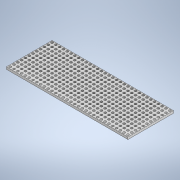
# Autodesk Inventor part: TamiyaUniversalPlate60-160
Saved by Autodesk Inventor 2022 (Build 260153000, 153)
## iProperties
Created: 2021-07-08
Part Number: TamiyaUniversalPlate60-160
Material: 一般
Document SubType Name: Modeling
Designer: ken
Density: 1 g/cm^3
Appearance: 既定
Author: ken
Autodesk Inventor part; units mm, degrees
ref_plane "YZ Plane" through (0, 0, 0) normal (1, 0, 0) x (0, 1, 0)
ref_plane "XZ Plane" through (0, 0, 0) normal (0, 1, 0) x (-1, 0, 0)
ref_plane "XY Plane" through (0, 0, 0) normal (0, 0, 1) x (1, 0, 0)
sketch "スケッチ1" plane through (0, 0, 0) normal (0, 1, 0) x (-1, 0, 0)
  line L0 (0, 0) -> (160, 0)
  line L1 (160, 0) -> (160, -60)
  line L2 (160, -60) -> (0, -60)
  line L3 (0, -60) -> (0, 0)
  dimension "d0" = 160
  dimension "d1" = 60
  constraints: 8 end point, 2 parallel, 1 horizontal, 1 perpendicular
  measures "d0" distance of L1.end L2.end
  measures "d1" distance of L0.end L1.end
extrude "押し出し1" add sketch "スケッチ1" along normal blind 3
sketch "スケッチ2" plane through (0, 3, 0) normal (0, 1, 0) x (1, 0, 0)
  line L0 (-160, 60) -> (-160, 0) projected
  line L1 (-160, 0) -> (0, 0) projected
  line L2 (0, 60) -> (-160, 60) projected
  line L3 (0, 0) -> (0, 60) projected
  point P0 (-77.5, 2.5)
  point P1 (-77.5, 7.5)
  point P2 (-77.5, 12.5)
  point P3 (-77.5, 17.5)
  point P4 (-77.5, 22.5)
  point P5 (-77.5, 27.5)
  point P6 (-77.5, 32.5)
  point P7 (-77.5, 37.5)
  point P8 (-77.5, 47.5)
  point P9 (-77.5, 42.5)
  point P10 (-77.5, 52.5)
  point P11 (-77.5, 57.5)
  point P12 (-72.5, 2.5)
  point P13 (-72.5, 7.5)
  point P14 (-72.5, 12.5)
  point P15 (-72.5, 17.5)
  point P16 (-72.5, 22.5)
  point P17 (-72.5, 27.5)
  point P18 (-72.5, 32.5)
  point P19 (-72.5, 37.5)
  point P20 (-72.5, 47.5)
  point P21 (-72.5, 42.5)
  point P22 (-72.5, 52.5)
  point P23 (-72.5, 57.5)
  point P24 (-67.5, 2.5)
  point P25 (-67.5, 7.5)
  point P26 (-67.5, 12.5)
  point P27 (-67.5, 17.5)
  point P28 (-67.5, 22.5)
  point P29 (-67.5, 27.5)
  point P30 (-67.5, 32.5)
  point P31 (-67.5, 37.5)
  point P32 (-67.5, 47.5)
  point P33 (-67.5, 42.5)
  point P34 (-67.5, 52.5)
  point P35 (-67.5, 57.5)
  point P36 (-62.5, 2.5)
  point P37 (-62.5, 7.5)
  point P38 (-62.5, 12.5)
  point P39 (-62.5, 17.5)
  point P40 (-62.5, 22.5)
  point P41 (-62.5, 27.5)
  point P42 (-62.5, 32.5)
  point P43 (-62.5, 37.5)
  point P44 (-62.5, 47.5)
  point P45 (-62.5, 42.5)
  point P46 (-62.5, 52.5)
  point P47 (-62.5, 57.5)
  point P48 (-57.5, 2.5)
  point P49 (-57.5, 7.5)
  point P50 (-57.5, 12.5)
  point P51 (-57.5, 17.5)
  point P52 (-57.5, 22.5)
  point P53 (-57.5, 27.5)
  point P54 (-57.5, 32.5)
  point P55 (-57.5, 37.5)
  point P56 (-57.5, 47.5)
  point P57 (-57.5, 42.5)
  point P58 (-57.5, 52.5)
  point P59 (-57.5, 57.5)
  point P60 (-52.5, 57.5)
  point P61 (-52.5, 52.5)
  point P62 (-52.5, 42.5)
  point P63 (-52.5, 47.5)
  point P64 (-52.5, 37.5)
  point P65 (-52.5, 32.5)
  point P66 (-52.5, 27.5)
  point P67 (-52.5, 22.5)
  point P68 (-52.5, 17.5)
  point P69 (-52.5, 12.5)
  point P70 (-52.5, 7.5)
  point P71 (-52.5, 2.5)
  point P72 (-47.5, 57.5)
  point P73 (-47.5, 52.5)
  point P74 (-47.5, 42.5)
  point P75 (-47.5, 47.5)
  point P76 (-47.5, 37.5)
  point P77 (-47.5, 32.5)
  point P78 (-47.5, 27.5)
  point P79 (-47.5, 22.5)
  point P80 (-47.5, 17.5)
  point P81 (-47.5, 12.5)
  point P82 (-47.5, 7.5)
  point P83 (-47.5, 2.5)
  point P84 (-42.5, 57.5)
  point P85 (-42.5, 52.5)
  point P86 (-42.5, 42.5)
  point P87 (-42.5, 47.5)
  point P88 (-42.5, 37.5)
  point P89 (-42.5, 32.5)
  point P90 (-42.5, 27.5)
  point P91 (-42.5, 22.5)
  point P92 (-42.5, 17.5)
  point P93 (-42.5, 12.5)
  point P94 (-42.5, 7.5)
  point P95 (-42.5, 2.5)
  point P96 (-37.5, 2.5)
  point P97 (-37.5, 7.5)
  point P98 (-37.5, 12.5)
  point P99 (-37.5, 17.5)
  point P100 (-37.5, 22.5)
  point P101 (-37.5, 27.5)
  point P102 (-37.5, 32.5)
  point P103 (-37.5, 37.5)
  point P104 (-37.5, 47.5)
  point P105 (-37.5, 42.5)
  point P106 (-37.5, 52.5)
  point P107 (-37.5, 57.5)
  point P108 (-32.5, 57.5)
  point P109 (-32.5, 52.5)
  point P110 (-32.5, 42.5)
  point P111 (-32.5, 47.5)
  point P112 (-32.5, 37.5)
  point P113 (-32.5, 32.5)
  point P114 (-32.5, 27.5)
  point P115 (-32.5, 22.5)
  point P116 (-32.5, 17.5)
  point P117 (-32.5, 12.5)
  point P118 (-32.5, 7.5)
  point P119 (-32.5, 2.5)
  point P120 (-27.5, 57.5)
  point P121 (-27.5, 52.5)
  point P122 (-27.5, 42.5)
  point P123 (-27.5, 47.5)
  point P124 (-27.5, 37.5)
  point P125 (-27.5, 32.5)
  point P126 (-27.5, 27.5)
  point P127 (-27.5, 22.5)
  point P128 (-27.5, 17.5)
  point P129 (-27.5, 12.5)
  point P130 (-27.5, 7.5)
  point P131 (-27.5, 2.5)
  point P132 (-22.5, 57.5)
  point P133 (-22.5, 52.5)
  point P134 (-22.5, 42.5)
  point P135 (-22.5, 47.5)
  point P136 (-22.5, 37.5)
  point P137 (-22.5, 32.5)
  point P138 (-22.5, 27.5)
  point P139 (-22.5, 22.5)
  point P140 (-22.5, 17.5)
  point P141 (-22.5, 12.5)
  point P142 (-22.5, 7.5)
  point P143 (-22.5, 2.5)
  point P144 (-17.5, 2.5)
  point P145 (-17.5, 7.5)
  point P146 (-17.5, 12.5)
  point P147 (-17.5, 17.5)
  point P148 (-17.5, 22.5)
  point P149 (-17.5, 27.5)
  point P150 (-17.5, 32.5)
  point P151 (-17.5, 37.5)
  point P152 (-17.5, 47.5)
  point P153 (-17.5, 42.5)
  point P154 (-17.5, 52.5)
  point P155 (-17.5, 57.5)
  point P156 (-12.5, 57.5)
  point P157 (-12.5, 52.5)
  point P158 (-12.5, 42.5)
  point P159 (-12.5, 47.5)
  point P160 (-12.5, 37.5)
  point P161 (-12.5, 32.5)
  point P162 (-12.5, 27.5)
  point P163 (-12.5, 22.5)
  point P164 (-12.5, 17.5)
  point P165 (-12.5, 12.5)
  point P166 (-12.5, 7.5)
  point P167 (-12.5, 2.5)
  point P168 (-7.5, 57.5)
  point P169 (-7.5, 52.5)
  point P170 (-7.5, 42.5)
  point P171 (-7.5, 47.5)
  point P172 (-7.5, 37.5)
  point P173 (-7.5, 32.5)
  point P174 (-7.5, 27.5)
  point P175 (-7.5, 22.5)
  point P176 (-7.5, 17.5)
  point P177 (-7.5, 12.5)
  point P178 (-7.5, 7.5)
  point P179 (-7.5, 2.5)
  point P180 (-2.5, 57.5)
  point P181 (-2.5, 52.5)
  point P182 (-2.5, 42.5)
  point P183 (-2.5, 47.5)
  point P184 (-2.5, 37.5)
  point P185 (-2.5, 32.5)
  point P186 (-2.5, 27.5)
  point P187 (-2.5, 22.5)
  point P188 (-2.5, 17.5)
  point P189 (-2.5, 12.5)
  point P190 (-2.5, 7.5)
  point P191 (-2.5, 2.5)
  point P192 (-157.5, 2.5)
  point P193 (-157.5, 7.5)
  point P194 (-157.5, 12.5)
  point P195 (-157.5, 17.5)
  point P196 (-157.5, 22.5)
  point P197 (-157.5, 27.5)
  point P198 (-157.5, 32.5)
  point P199 (-157.5, 37.5)
  dimension "d4" = 5
  dimension "d5" = 2.5
  dimension "d6" = 5
  dimension "d7" = 5
  dimension "d8" = 5
  dimension "d9" = 5
  dimension "d10" = 5
  dimension "d11" = 5
  dimension "d12" = 5
  dimension "d13" = 5
  dimension "d14" = 5
  dimension "d15" = 5
  dimension "d16" = 2.5
  dimension "d17" = 2.5
  dimension "d18" = 5
  dimension "d19" = 5
  dimension "d20" = 5
  dimension "d21" = 5
  dimension "d22" = 5
  dimension "d23" = 5
  dimension "d24" = 5
  dimension "d25" = 5
  dimension "d26" = 5
  dimension "d27" = 5
  dimension "d28" = 5
  dimension "d29" = 5
  dimension "d30" = 5
  dimension "d31" = 5
  dimension "d32" = 5
  dimension "d33" = 5
  dimension "d34" = 5
  dimension "d35" = 5
  dimension "d36" = 5
  dimension "d37" = 5
  dimension "d38" = 5
  dimension "d39" = 5
  dimension "d40" = 5
  dimension "d41" = 5
  dimension "d42" = 5
  dimension "d43" = 5
  dimension "d44" = 5
  dimension "d45" = 5
  dimension "d46" = 5
  dimension "d47" = 5
  dimension "d48" = 5
  dimension "d49" = 5
  dimension "d50" = 5
  dimension "d51" = 5
  dimension "d52" = 5
  dimension "d53" = 5
  dimension "d54" = 5
  dimension "d55" = 5
  dimension "d56" = 5
  dimension "d57" = 5
  dimension "d58" = 5
  dimension "d59" = 5
  dimension "d60" = 5
  dimension "d61" = 5
  dimension "d62" = 5
  dimension "d63" = 5
  dimension "d64" = 5
  dimension "d65" = 5
  dimension "d66" = 5
  dimension "d67" = 5
  constraints: 352 vertical alignment, 24 horizontal alignment
  measures "d4" distance of point (-77.5, 2.5) point (-77.5, 7.5)
  measures "d6" distance of point (-77.5, 7.5) point (-77.5, 12.5)
  measures "d7" distance of point (-77.5, 12.5) point (-77.5, 17.5)
  measures "d8" distance of point (-77.5, 17.5) point (-77.5, 22.5)
  measures "d9" distance of point (-77.5, 22.5) point (-77.5, 27.5)
  measures "d10" distance of point (-77.5, 27.5) point (-77.5, 32.5)
  measures "d11" distance of point (-77.5, 37.5) point (-77.5, 32.5)
  measures "d12" distance of point (-77.5, 42.5) point (-77.5, 37.5)
  measures "d13" distance of point (-77.5, 47.5) point (-77.5, 42.5)
  measures "d14" distance of point (-77.5, 52.5) point (-77.5, 47.5)
  measures "d15" distance of point (-77.5, 57.5) point (-77.5, 52.5)
  measures "d16" distance from line of L1 point (-77.5, 2.5)
  measures "d17" distance from line of L2 point (-77.5, 57.5)
  measures "d18" distance of point (-72.5, 2.5) point (-72.5, 7.5)
  measures "d19" distance of point (-72.5, 7.5) point (-72.5, 12.5)
  measures "d20" distance of point (-72.5, 12.5) point (-72.5, 17.5)
  measures "d21" distance of point (-72.5, 17.5) point (-72.5, 22.5)
  measures "d22" distance of point (-72.5, 22.5) point (-72.5, 27.5)
  measures "d23" distance of point (-72.5, 27.5) point (-72.5, 32.5)
  measures "d24" distance of point (-72.5, 37.5) point (-72.5, 32.5)
  measures "d25" distance of point (-72.5, 42.5) point (-72.5, 37.5)
  measures "d26" distance of point (-72.5, 47.5) point (-72.5, 42.5)
  measures "d27" distance of point (-72.5, 52.5) point (-72.5, 47.5)
  measures "d28" distance of point (-72.5, 57.5) point (-72.5, 52.5)
  measures "d29" distance of point (-67.5, 2.5) point (-67.5, 7.5)
  measures "d30" distance of point (-67.5, 7.5) point (-67.5, 12.5)
  measures "d31" distance of point (-67.5, 12.5) point (-67.5, 17.5)
  measures "d32" distance of point (-67.5, 17.5) point (-67.5, 22.5)
  measures "d33" distance of point (-67.5, 22.5) point (-67.5, 27.5)
  measures "d34" distance of point (-67.5, 27.5) point (-67.5, 32.5)
  measures "d35" distance of point (-67.5, 37.5) point (-67.5, 32.5)
  measures "d36" distance of point (-67.5, 42.5) point (-67.5, 37.5)
  measures "d37" distance of point (-67.5, 47.5) point (-67.5, 42.5)
  measures "d38" distance of point (-67.5, 52.5) point (-67.5, 47.5)
  measures "d39" distance of point (-67.5, 57.5) point (-67.5, 52.5)
  measures "d40" distance of point (-62.5, 2.5) point (-62.5, 7.5)
  measures "d41" distance of point (-62.5, 7.5) point (-62.5, 12.5)
  measures "d42" distance of point (-62.5, 12.5) point (-62.5, 17.5)
  measures "d43" distance of point (-62.5, 17.5) point (-62.5, 22.5)
  measures "d44" distance of point (-62.5, 22.5) point (-62.5, 27.5)
  measures "d45" distance of point (-62.5, 27.5) point (-62.5, 32.5)
  measures "d46" distance of point (-62.5, 37.5) point (-62.5, 32.5)
  measures "d47" distance of point (-62.5, 42.5) point (-62.5, 37.5)
  measures "d48" distance of point (-62.5, 47.5) point (-62.5, 42.5)
  measures "d49" distance of point (-62.5, 52.5) point (-62.5, 47.5)
  measures "d50" distance of point (-62.5, 57.5) point (-62.5, 52.5)
  measures "d51" distance of point (-77.5, 2.5) point (-72.5, 2.5)
  measures "d52" distance of point (-72.5, 2.5) point (-67.5, 2.5)
  measures "d53" distance of point (-67.5, 2.5) point (-62.5, 2.5)
  measures "d54" distance of point (-57.5, 2.5) point (-57.5, 7.5)
  measures "d55" distance of point (-57.5, 7.5) point (-57.5, 12.5)
  measures "d56" distance of point (-57.5, 12.5) point (-57.5, 17.5)
  measures "d57" distance of point (-57.5, 17.5) point (-57.5, 22.5)
  measures "d58" distance of point (-57.5, 22.5) point (-57.5, 27.5)
  measures "d59" distance of point (-57.5, 27.5) point (-57.5, 32.5)
  measures "d60" distance of point (-57.5, 37.5) point (-57.5, 32.5)
  measures "d61" distance of point (-57.5, 42.5) point (-57.5, 37.5)
  measures "d62" distance of point (-57.5, 47.5) point (-57.5, 42.5)
  measures "d63" distance of point (-57.5, 52.5) point (-57.5, 47.5)
  measures "d64" distance of point (-57.5, 57.5) point (-57.5, 52.5)
  measures "d65" distance of point (-52.5, 2.5) point (-52.5, 7.5)
  measures "d66" distance of point (-52.5, 7.5) point (-52.5, 12.5)
  measures "d67" distance of point (-52.5, 12.5) point (-52.5, 17.5)
hole "穴1" at (-157.5, 3, -2.5) at (-157.5, 3, -7.5) at (-157.5, 3, -12.5) at (-157.5, 3, -17.5) at (-157.5, 3, -22.5) at (-157.5, 3, -27.5) at (-157.5, 3, -32.5) at (-157.5, 3, -37.5) at (-157.5, 3, -47.5) at (-157.5, 3, -42.5) at (-157.5, 3, -52.5) at (-157.5, 3, -57.5) at (-152.5, 3, -57.5) at (-152.5, 3, -52.5) at (-152.5, 3, -42.5) at (-152.5, 3, -47.5) at (-152.5, 3, -37.5) at (-152.5, 3, -32.5) at (-152.5, 3, -27.5) at (-152.5, 3, -22.5) at (-152.5, 3, -17.5) at (-152.5, 3, -12.5) at (-152.5, 3, -7.5) at (-152.5, 3, -2.5) at (-147.5, 3, -57.5) at (-147.5, 3, -52.5) at (-147.5, 3, -42.5) at (-147.5, 3, -47.5) at (-147.5, 3, -37.5) at (-147.5, 3, -32.5) at (-147.5, 3, -27.5) at (-147.5, 3, -22.5) at (-147.5, 3, -17.5) at (-147.5, 3, -12.5) at (-147.5, 3, -7.5) at (-147.5, 3, -2.5) at (-142.5, 3, -57.5) at (-142.5, 3, -52.5) at (-142.5, 3, -42.5) at (-142.5, 3, -47.5) at (-142.5, 3, -37.5) at (-142.5, 3, -32.5) at (-142.5, 3, -27.5) at (-142.5, 3, -22.5) at (-142.5, 3, -17.5) at (-142.5, 3, -12.5) at (-142.5, 3, -7.5) at (-142.5, 3, -2.5) at (-122.5, 3, -2.5) at (-122.5, 3, -7.5) direction (0, -1, 0) diameter 3 depth 3 and at (-122.5, 3, -12.5) (-122.5, 3, -17.5) (-122.5, 3, -22.5) (-122.5, 3, -27.5) (-122.5, 3, -32.5) (-122.5, 3, -37.5) (-122.5, 3, -47.5) (-122.5, 3, -42.5) (-122.5, 3, -52.5) (-122.5, 3, -57.5) (-127.5, 3, -2.5) (-127.5, 3, -7.5) (-127.5, 3, -12.5) (-127.5, 3, -17.5) (-127.5, 3, -22.5) (-127.5, 3, -27.5) (-127.5, 3, -32.5) (-127.5, 3, -37.5) (-127.5, 3, -47.5) (-127.5, 3, -42.5) (-127.5, 3, -52.5) (-127.5, 3, -57.5) (-132.5, 3, -2.5) (-132.5, 3, -7.5) (-132.5, 3, -12.5) (-132.5, 3, -17.5) (-132.5, 3, -22.5) (-132.5, 3, -27.5) (-132.5, 3, -32.5) (-132.5, 3, -37.5) (-132.5, 3, -47.5) (-132.5, 3, -42.5) (-132.5, 3, -52.5) (-132.5, 3, -57.5) (-137.5, 3, -57.5) (-137.5, 3, -52.5) (-137.5, 3, -42.5) (-137.5, 3, -47.5) (-137.5, 3, -37.5) (-137.5, 3, -32.5) (-137.5, 3, -27.5) (-137.5, 3, -22.5) (-137.5, 3, -17.5) (-137.5, 3, -12.5) (-137.5, 3, -7.5) (-137.5, 3, -2.5) (-102.5, 3, -2.5) (-102.5, 3, -7.5) (-102.5, 3, -12.5) (-102.5, 3, -17.5) (-102.5, 3, -22.5) (-102.5, 3, -27.5) (-102.5, 3, -32.5) (-102.5, 3, -37.5) (-102.5, 3, -47.5) (-102.5, 3, -42.5) (-102.5, 3, -52.5) (-102.5, 3, -57.5) (-107.5, 3, -2.5) (-107.5, 3, -7.5) (-107.5, 3, -12.5) (-107.5, 3, -17.5) (-107.5, 3, -22.5) (-107.5, 3, -27.5) (-107.5, 3, -32.5) (-107.5, 3, -37.5) (-107.5, 3, -47.5) (-107.5, 3, -42.5) (-107.5, 3, -52.5) (-107.5, 3, -57.5) (-112.5, 3, -2.5) (-112.5, 3, -7.5) (-112.5, 3, -12.5) (-112.5, 3, -17.5) (-112.5, 3, -22.5) (-112.5, 3, -27.5) (-112.5, 3, -32.5) (-112.5, 3, -37.5) (-112.5, 3, -47.5) (-112.5, 3, -42.5) (-112.5, 3, -52.5) (-112.5, 3, -57.5) (-117.5, 3, -57.5) (-117.5, 3, -52.5) (-117.5, 3, -42.5) (-117.5, 3, -47.5) (-117.5, 3, -37.5) (-117.5, 3, -32.5) (-117.5, 3, -27.5) (-117.5, 3, -22.5) (-117.5, 3, -17.5) (-117.5, 3, -12.5) (-117.5, 3, -7.5) (-117.5, 3, -2.5) (-82.5, 3, -2.5) (-82.5, 3, -7.5) (-82.5, 3, -12.5) (-82.5, 3, -17.5) (-82.5, 3, -22.5) (-82.5, 3, -27.5) (-82.5, 3, -32.5) (-82.5, 3, -37.5) (-82.5, 3, -47.5) (-82.5, 3, -42.5) (-82.5, 3, -52.5) (-82.5, 3, -57.5) (-87.5, 3, -2.5) (-87.5, 3, -7.5) (-87.5, 3, -12.5) (-87.5, 3, -17.5) (-87.5, 3, -22.5) (-87.5, 3, -27.5) (-87.5, 3, -32.5) (-87.5, 3, -37.5) (-87.5, 3, -47.5) (-87.5, 3, -42.5) (-87.5, 3, -52.5) (-87.5, 3, -57.5) (-92.5, 3, -2.5) (-92.5, 3, -7.5) (-92.5, 3, -12.5) (-92.5, 3, -17.5) (-92.5, 3, -22.5) (-92.5, 3, -27.5) (-92.5, 3, -32.5) (-92.5, 3, -37.5) (-92.5, 3, -47.5) (-92.5, 3, -42.5) (-92.5, 3, -52.5) (-92.5, 3, -57.5) (-97.5, 3, -57.5) (-97.5, 3, -52.5) (-97.5, 3, -42.5) (-97.5, 3, -47.5) (-97.5, 3, -37.5) (-97.5, 3, -32.5) (-97.5, 3, -27.5) (-97.5, 3, -22.5) (-97.5, 3, -17.5) (-97.5, 3, -12.5) (-97.5, 3, -7.5) (-97.5, 3, -2.5) (-17.5, 3, -2.5) (-17.5, 3, -7.5) (-17.5, 3, -12.5) (-17.5, 3, -17.5) (-17.5, 3, -22.5) (-17.5, 3, -27.5) (-17.5, 3, -32.5) (-17.5, 3, -37.5) (-17.5, 3, -47.5) (-17.5, 3, -42.5) (-17.5, 3, -52.5) (-17.5, 3, -57.5) (-12.5, 3, -57.5) (-12.5, 3, -52.5) (-12.5, 3, -42.5) (-12.5, 3, -47.5) (-12.5, 3, -37.5) (-12.5, 3, -32.5) (-12.5, 3, -27.5) (-12.5, 3, -22.5) (-12.5, 3, -17.5) (-12.5, 3, -12.5) (-12.5, 3, -7.5) (-12.5, 3, -2.5) (-7.5, 3, -57.5) (-7.5, 3, -52.5) (-7.5, 3, -42.5) (-7.5, 3, -47.5) (-7.5, 3, -37.5) (-7.5, 3, -32.5) (-7.5, 3, -27.5) (-7.5, 3, -22.5) (-7.5, 3, -17.5) (-7.5, 3, -12.5) (-7.5, 3, -7.5) (-7.5, 3, -2.5) (-2.5, 3, -57.5) (-2.5, 3, -52.5) (-2.5, 3, -42.5) (-2.5, 3, -47.5) (-2.5, 3, -37.5) (-2.5, 3, -32.5) (-2.5, 3, -27.5) (-2.5, 3, -22.5) (-2.5, 3, -17.5) (-2.5, 3, -12.5) (-2.5, 3, -7.5) (-2.5, 3, -2.5) (-37.5, 3, -2.5) (-37.5, 3, -7.5) (-37.5, 3, -12.5) (-37.5, 3, -17.5) (-37.5, 3, -22.5) (-37.5, 3, -27.5) (-37.5, 3, -32.5) (-37.5, 3, -37.5) (-37.5, 3, -47.5) (-37.5, 3, -42.5) (-37.5, 3, -52.5) (-37.5, 3, -57.5) (-32.5, 3, -57.5) (-32.5, 3, -52.5) (-32.5, 3, -42.5) (-32.5, 3, -47.5) (-32.5, 3, -37.5) (-32.5, 3, -32.5) (-32.5, 3, -27.5) (-32.5, 3, -22.5) (-32.5, 3, -17.5) (-32.5, 3, -12.5) (-32.5, 3, -7.5) (-32.5, 3, -2.5) (-27.5, 3, -57.5) (-27.5, 3, -52.5) (-27.5, 3, -42.5) (-27.5, 3, -47.5) (-27.5, 3, -37.5) (-27.5, 3, -32.5) (-27.5, 3, -27.5) (-27.5, 3, -22.5) (-27.5, 3, -17.5) (-27.5, 3, -12.5) (-27.5, 3, -7.5) (-27.5, 3, -2.5) (-22.5, 3, -57.5) (-22.5, 3, -52.5) (-22.5, 3, -42.5) (-22.5, 3, -47.5) (-22.5, 3, -37.5) (-22.5, 3, -32.5) (-22.5, 3, -27.5) (-22.5, 3, -22.5) (-22.5, 3, -17.5) (-22.5, 3, -12.5) (-22.5, 3, -7.5) (-22.5, 3, -2.5) (-57.5, 3, -2.5) (-57.5, 3, -7.5) (-57.5, 3, -12.5) (-57.5, 3, -17.5) (-57.5, 3, -22.5) (-57.5, 3, -27.5) (-57.5, 3, -32.5) (-57.5, 3, -37.5) (-57.5, 3, -47.5) (-57.5, 3, -42.5) (-57.5, 3, -52.5) (-57.5, 3, -57.5) (-52.5, 3, -57.5) (-52.5, 3, -52.5) (-52.5, 3, -42.5) (-52.5, 3, -47.5) (-52.5, 3, -37.5) (-52.5, 3, -32.5) (-52.5, 3, -27.5) (-52.5, 3, -22.5) (-52.5, 3, -17.5) (-52.5, 3, -12.5) (-52.5, 3, -7.5) (-52.5, 3, -2.5) (-47.5, 3, -57.5) (-47.5, 3, -52.5) (-47.5, 3, -42.5) (-47.5, 3, -47.5) (-47.5, 3, -37.5) (-47.5, 3, -32.5) (-47.5, 3, -27.5) (-47.5, 3, -22.5) (-47.5, 3, -17.5) (-47.5, 3, -12.5) (-47.5, 3, -7.5) (-47.5, 3, -2.5) (-42.5, 3, -57.5) (-42.5, 3, -52.5) (-42.5, 3, -42.5) (-42.5, 3, -47.5) (-42.5, 3, -37.5) (-42.5, 3, -32.5) (-42.5, 3, -27.5) (-42.5, 3, -22.5) (-42.5, 3, -17.5) (-42.5, 3, -12.5) (-42.5, 3, -7.5) (-42.5, 3, -2.5) (-62.5, 3, -2.5) (-62.5, 3, -7.5) (-62.5, 3, -12.5) (-62.5, 3, -17.5) (-62.5, 3, -22.5) (-62.5, 3, -27.5) (-62.5, 3, -32.5) (-62.5, 3, -37.5) (-62.5, 3, -47.5) (-62.5, 3, -42.5) (-62.5, 3, -52.5) (-62.5, 3, -57.5) (-67.5, 3, -2.5) (-67.5, 3, -7.5) (-67.5, 3, -12.5) (-67.5, 3, -17.5) (-67.5, 3, -22.5) (-67.5, 3, -27.5) (-67.5, 3, -32.5) (-67.5, 3, -37.5) (-67.5, 3, -47.5) (-67.5, 3, -42.5) (-67.5, 3, -52.5) (-67.5, 3, -57.5) (-72.5, 3, -2.5) (-72.5, 3, -7.5) (-72.5, 3, -12.5) (-72.5, 3, -17.5) (-72.5, 3, -22.5) (-72.5, 3, -27.5) (-72.5, 3, -32.5) (-72.5, 3, -37.5) (-72.5, 3, -47.5) (-72.5, 3, -42.5) (-72.5, 3, -52.5) (-72.5, 3, -57.5) (-77.5, 3, -57.5) (-77.5, 3, -52.5) (-77.5, 3, -42.5) (-77.5, 3, -47.5) (-77.5, 3, -37.5) (-77.5, 3, -32.5) (-77.5, 3, -27.5) (-77.5, 3, -22.5) (-77.5, 3, -17.5) (-77.5, 3, -12.5) (-77.5, 3, -7.5) (-77.5, 3, -2.5)
